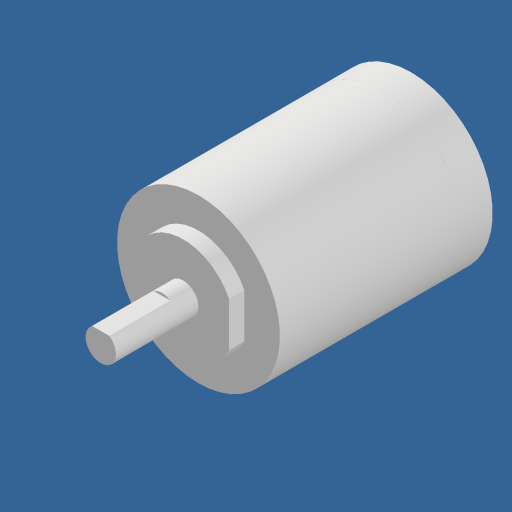
# Autodesk Inventor part: PlanetaryGearbox
Saved by Autodesk Inventor 2023 (Build 270158030, 158C)
## iProperties
Created: 2023-02-26
Part Number: PlanetaryGearbox
Material: Generic
Document SubType Name: Modeling
Designer: kumpu
Density: 1 g/cm^3
Appearance: Default
Author: kumpu
Autodesk Inventor part; units mm, degrees
ref_plane "YZ Plane" through (0, 0, 0) normal (1, 0, 0) x (0, 1, 0)
ref_plane "XZ Plane" through (0, 0, 0) normal (0, 1, 0) x (-1, 0, 0)
ref_plane "XY Plane" through (0, 0, 0) normal (0, 0, 1) x (1, 0, 0)
sketch "Sketch1" plane through (0, 0, 0) normal (1, 0, 0) x (0, 1, 0)
  line L0 (0, 61) -> (3, 61)
  line L1 (3, 61) -> (3, 44.8)
  line L2 (3, 44.8) -> (10, 44.8)
  line L3 (10, 44.8) -> (10, 41.8)
  line L4 (10, 41.8) -> (16, 41.8)
  line L5 (16, 41.8) -> (16, 35.8)
  line L6 (16, 35.8) -> (15.99, 35.8)
  line L7 (15.99, 35.8) -> (15.99, 6)
  line L8 (15.99, 6) -> (16, 6)
  line L9 (16, 6) -> (16, 0)
  line L10 (16, 0) -> (0, 0)
  line L11 (0, 0) -> (0, 61)
  point P0 (1.5, 61)
  dimension "d0" = 6
  dimension "d1" = 32
  dimension "d2" = 6
  dimension "d3" = 19.2
  dimension "d4" = 41.8
  dimension "d5" = 3
  dimension "d6" = 20
  dimension "d7" = 0.01
  constraints: 24 end point, 10 perpendicular, 2 point on line, 1 coincident, 1 collinear, 1 midpoint, 1 vertical
  measures "d0" diameter of L1 L11
  measures "d1" diameter of L5 L11
  measures "d2" distance of L8.end L9.end
  measures "d3" distance from line of point (1.5, 61) L4
  measures "d4" distance between parallel lines of L4 L10
  measures "d5" distance of L2.end L3.end
  measures "d6" diameter of L3 L11
  measures "d7" distance of L5.end L6.end
revolve "Revolution1" add sketch "Sketch1" angle 360 about axis through (0, 0, 0) along (0, 0, 1)
sketch "Sketch2" plane through (0, 0, 61) normal (0, 0, 1) x (1, 0, 0)
  arc A0 (1.6583, 2.5) -> (-1.6583, 2.5) centre (0, 0) ccw
  line L0 (-1.6583, 2.5) -> (1.6583, 2.5)
  circle A1 centre (0, 0) radius 3 projected
  dimension "d9" = 2.5
  constraints: 2 concentric, 2 end point, 2 point on circle, 1 centre point, 1 horizontal
  measures "d9" distance from line of A0.centre L0
extrude "Extrusion1" cut sketch "Sketch2" against normal blind 12 contours L0 A0
sketch "Sketch3" plane through (0, 0, 44.8) normal (0, 0, 1) x (1, 0, 0)
  line L0 (-9, 4.3589) -> (-9, -4.3589)
  line L1 (9, 4.3589) -> (9, -4.3589)
  arc A0 (-9, 4.3589) -> (-9, -4.3589) centre (0, 0) ccw
  arc A1 (9, -4.3589) -> (9, 4.3589) centre (0, 0) ccw
  circle A2 centre (0, 0) radius 10 construction
  dimension "d12" = 18
  constraints: 4 concentric, 4 end point, 4 point on circle, 2 centre point, 2 vertical, 1 parallel
  measures "d12" distance between parallel lines of L0 L1
extrude "Extrusion2" cut sketch "Sketch3" against normal up to surface (3 mm away)
body "Solid1"
